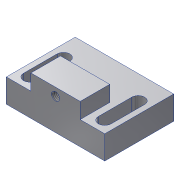
# Autodesk Inventor part: Clamping Block
Saved by Autodesk Inventor 2016 (Build 200138000, 138)
## iProperties
Created: 2015-08-18
Part Number: Clamping Block
Material: Aluminum 6061
Document SubType Name: Modeling
Density: 2.7 g/cm^3
Appearance: Aluminum - Flat
Autodesk Inventor part; units mm, degrees
ref_plane "YZ Plane" through (0, 0, 0) normal (1, 0, 0) x (0, 1, 0)
ref_plane "XZ Plane" through (0, 0, 0) normal (0, 1, 0) x (-1, 0, 0)
ref_plane "XY Plane" through (0, 0, 0) normal (0, 0, 1) x (1, 0, 0)
sketch "Sketch1" plane through (0, 0, 0) normal (1, 0, 0) x (0, 1, 0)
  line L0 (0, 20) -> (15, 20)
  line L1 (15, 20) -> (15, 12)
  line L2 (15, 12) -> (35, 12)
  line L3 (35, 12) -> (35, 0)
  line L4 (35, 0) -> (0, 0)
  line L5 (0, 0) -> (0, 20)
  dimension "d0" = 35
  dimension "d30" = 20
  dimension "d31" = 8
  dimension "d33" = 20
  constraints: 12 end point, 4 perpendicular, 1 coincident, 1 horizontal
  measures "d0" distance between parallel lines of L5 L3
  measures "d30" distance between parallel lines of L3 L1
  measures "d31" distance between parallel lines of L0 L2
  measures "d33" distance between parallel lines of L0 L4
extrude "Extrusion1" add sketch "Sketch1" along normal mid plane 50
sketch "Sketch2" plane through (-25, 0, 0) normal (0, -1, 0) x (1, 0, 0)
  line L0 (0, 20) -> (12.5, 20)
  line L1 (12.5, 20) -> (12.5, 12)
  line L2 (12.5, 12) -> (0, 12)
  line L3 (0, 12) -> (0, 20)
  line L4 (37.5, 20) -> (50, 20)
  line L5 (50, 20) -> (50, 12)
  line L6 (50, 12) -> (37.5, 12)
  line L7 (37.5, 12) -> (37.5, 20)
  line L8 (0, 20) -> (50, 20) projected
  line L9 (50, 12) -> (0, 12) projected
  dimension "d15" = 25
  constraints: 16 end point, 4 parallel, 3 collinear, 2 horizontal, 2 perpendicular, 2 point on line
  measures "d15" distance between parallel lines of L7 L1
extrude "Extrusion2" cut sketch "Sketch2" against normal through all contours L0 L1 L2 L3 | L4 L5 L6 L7
sketch "Sketch4" plane through (-25, 35, 12) normal (0, 0, 1) x (1, 0, 0)
  line L0 (6, -29) -> (6, -12) construction
  line L1 (9.25, -29) -> (9.25, -12)
  line L2 (2.75, -12) -> (2.75, -29)
  arc A0 (2.75, -29) -> (9.25, -29) centre (6, -29) ccw
  arc A1 (9.25, -12) -> (2.75, -12) centre (6, -12) ccw
  line L3 (12.5, -35) -> (0, -35) projected
  line L4 (0, -35) -> (0, 0) projected
  point P0 (6, -20.5)
  dimension "d24" = 6.5
  dimension "d25" = 17
  dimension "d38" = 6
  dimension "d39" = 6
  constraints: 8 end point, 4 point on circle, 4 tangent, 2 centre point, 1 midpoint, 1 parallel, 1 vertical
  measures "d24" distance between parallel lines of L1 L2
  measures "d25" distance of L0.start L0.end
  measures "d38" distance from line of L3 L0.start
  measures "d39" distance between parallel lines of L0 L4
extrude "Extrusion3" cut sketch "Sketch4" against normal through all
mirror "Mirror1" about plane through (0, 0, 0) normal (1, 0, 0) of "Extrusion3"
sketch "Sketch5" plane through (-25, 0, 0) normal (0, -1, 0) x (1, 0, 0)
  line L0 (12.5, 20) -> (37.5, 20) projected
  point P0 (25, 0)
  point P1 (25, 16)
  point P2 (25, 20)
  dimension "d40" = 4
  constraints: 1 midpoint, 1 vertical alignment
  measures "d40" distance from line of L0 point (25, 16)
hole "Hole1" at (0, 0, 16) direction (0, 1, 0) diameter 4.134 end through all thread size "M5x0.8" designation "M5" class "6H" standard "ISO Metric profile"
body "Solid1"
